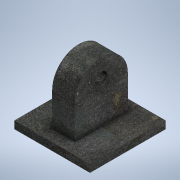
# Autodesk Inventor part: 02_10 Soporte01
Saved by Autodesk Inventor 2021 (Build 250183000, 183)
## iProperties
Created: 2021-06-25
Part Number: 02_10 Soporte01
Material: Acero ASTM A36
Document SubType Name: Modeling
Designer: Almanzor
Density: 7.85 g/cm^3
Appearance: Placa
Author: Almanzor
Autodesk Inventor part; units mm, degrees
ref_plane "YZ Plane" through (0, 0, 0) normal (1, 0, 0) x (0, 1, 0)
ref_plane "XZ Plane" through (0, 0, 0) normal (0, 1, 0) x (-1, 0, 0)
ref_plane "XY Plane" through (0, 0, 0) normal (0, 0, 1) x (1, 0, 0)
sketch "Boceto1" plane through (0, 0, 0) normal (0, 1, 0) x (-1, 0, 0)
  line L0 (50, 50) -> (-50, 50)
  line L1 (-50, 50) -> (-50, -50)
  line L2 (-50, -50) -> (50, -50)
  line L3 (50, -50) -> (50, 50)
  line L4 (50, 50) -> (-50, -50) construction
  line L5 (-50, 50) -> (50, -50) construction
  point P0 (0, 0)
  dimension "d0" = 100
  dimension "d1" = 100
  constraints: 12 end point, 2 midpoint, 2 parallel, 1 horizontal, 1 perpendicular
  measures "d0" distance of L1.end L2.end
  measures "d1" distance of L0.end L1.end
extrude "Extrusión1" add sketch "Boceto1" along normal blind 10
sketch "Boceto2" plane through (0, 10, 0) normal (0, 1, 0) x (1, 0, 0)
  line L0 (-15, 35) -> (15, 35)
  line L1 (15, 35) -> (15, -35)
  line L2 (15, -35) -> (-15, -35)
  line L3 (-15, -35) -> (-15, 35)
  line L4 (-15, 35) -> (15, -35) construction
  line L5 (15, 35) -> (-15, -35) construction
  point P0 (0, 0)
  dimension "d4" = 70
  dimension "d5" = 30
  constraints: 12 end point, 2 midpoint, 2 parallel, 1 horizontal, 1 perpendicular
  measures "d4" distance of L0.end L1.end
  measures "d5" distance of L1.end L2.end
extrude "Extrusión2" add sketch "Boceto2" along normal blind 80
sketch "Boceto3" plane through (-15, 10, -35) normal (-1, 0, 0) x (0, 0, 1)
  circle A0 centre (35, 55) radius 8.5
  line L0 (0, 0) -> (0, 80) projected
  line L1 (0, 80) -> (70, 80) projected
  point P0 (35, -10)
  dimension "d8" = 17
  dimension "d9" = 35
  dimension "d10" = 25
  constraints: 1 centre point
  measures "d8" diameter of A0
  measures "d9" distance from line of L0 A0.centre
  measures "d10" distance from line of L1 A0.centre
extrude "Extrusión3" cut sketch "Boceto3" along normal mid plane 80
fillet "Empalme1" radius 35 1 edges at (0, 90, -35)
fillet "Empalme2" radius 35 1 edges at (0, 90, 35)
